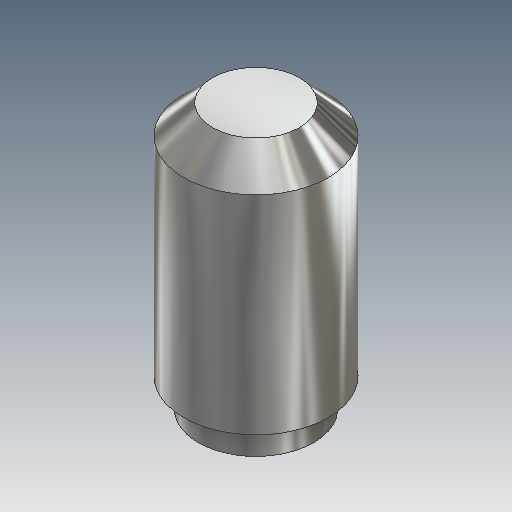
# Autodesk Inventor part: 00_Microscope_Objective_Lens10x
Saved by Autodesk Inventor 2019.4 (Build 234330000, 330)
## iProperties
Created: 2018-08-22
Part Number: 00_Microscope_Objective_Lens10x
Material: Generisch
Document SubType Name: Modeling
Designer: diederichbenedict
Density: 1 g/cm^3
Appearance: Chrom - poliert
Author: diederichbenedict
Autodesk Inventor part; units mm, degrees
ref_plane "YZ Plane" through (0, 0, 0) normal (1, 0, 0) x (0, 1, 0)
ref_plane "XZ Plane" through (0, 0, 0) normal (0, 1, 0) x (-1, 0, 0)
sketch "Skizze1" plane through (0, 0, 0) normal (0, 0, 1) x (1, 0, 0)
  circle A0 centre (-0.7274, 0.5828) radius 13
  circle A1 centre (-0.7274, 0.5828) radius 12.5
  dimension "d8" = 25
  constraints: 2 centre point, 1 coincident, 2 other
  measures "d8" diameter of A1
ref_plane "Arbeitsebene1" through (-32.0071, -13.4173, 43.0224) normal (0, 0, 1) x (0.7071, 0.7071, 0)
extrude "Extrusion1" add sketch "Skizze1" along normal blind 41 contours A1
chamfer "Fase1" distance 5 angle 45 1 edges at (-13.2274, 0.5828, 41)
sketch "Sketch2" plane through (-0.7274, 0.5828, 0) normal (0, 0, -1) x (-1, 0, 0)
  circle A0 centre (0, 0) radius 8.6364 projected
  circle A1 centre (0, 0) radius 13.6364 projected
  circle A2 centre (0, 0) radius 13.6364 projected
  circle A3 centre (0, 0) radius 10
  point P0 (-0.7274, -0.5828)
  dimension "d5" = 20
  constraints: 1 centre point, 1 coincident
  measures "d5" diameter of A3
extrude "Extrusion2" add sketch "Sketch2" along normal blind 5 contours A0 | A3
